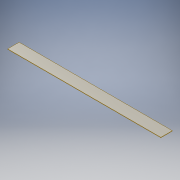
# Autodesk Inventor part: 導電性布
Saved by Autodesk Inventor 2019.4 (Build 234330000, 330)
## iProperties
Created: 2020-01-02
Part Number: 導電性布
Material: チタン
Document SubType Name: Modeling
Designer: Hideto Niwa
Density: 4.51 g/cm^3
Appearance: チタン
Author: Hideto Niwa
Autodesk Inventor part; units mm, degrees
ref_plane "YZ Plane" through (0, 0, 0) normal (1, 0, 0) x (0, 1, 0)
ref_plane "XZ Plane" through (0, 0, 0) normal (0, 1, 0) x (-1, 0, 0)
ref_plane "XY Plane" through (0, 0, 0) normal (0, 0, 1) x (1, 0, 0)
sketch "スケッチ1" plane through (0, 0, 0) normal (0, 1, 0) x (-1, 0, 0)
  line L0 (0, 0) -> (-200, 0)
  line L1 (-200, 0) -> (-200, -15)
  line L2 (-200, -15) -> (0, -15)
  line L3 (0, -15) -> (0, 0)
  dimension "d2" = 200
  dimension "d3" = 15
  constraints: 8 end point, 2 parallel, 1 horizontal, 1 perpendicular
  measures "d2" distance between parallel lines of L1 L3
  measures "d3" distance between parallel lines of L0 L2
extrude "押し出し1" add sketch "スケッチ1" along normal blind 0.5
